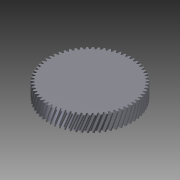
# Autodesk Inventor part: LargeGear
Saved by Autodesk Inventor 2012 (Build 160160000, 160)
## iProperties
Created: 2011-10-22
Part Number: LargeGear
Material: Steel
Document SubType Name: Modeling
Designer: KuttaA
Categories: <?xml version="1.0" encoding="UTF-16"?> <MemberInstance><Categories><FamilyTemplate><FamilyTemplateParameter ValueType="xs:double" Id="1" ObjectReferenceKey="da_z" ObjectType="kUserParameterObject"/><FamilyTemplateParameter ValueType="xs:double" Id="2" ObjectReferenceKey="da_b" ObjectType="kUserParameterObject"/><FamilyTemplateParameter ValueType="xs:double" Id="3" ObjectReferenceKey="da_beta" ObjectType="kUserParameterObject"/><FamilyTemplateParameter ValueType="xs:double" Id="4" ObjectReferenceKey="da_da" ObjectType="kUserParameterObject"/><FamilyTemplateParameter ValueType="xs:double" Id="5" ObjectReferenceKey="da_aw" ObjectType="kUserParameterObject"/><FamilyTemplateParameter ValueType="xs:string" Id="6" ObjectReferenceKey="EAIAABAAAACIAQAAAAAAAIAAAAAAAAAA" ObjectType="83910656" SubObjectId="SurfaceGeometry"/></FamilyTemplate><ParamToTemplateMap><ParamToTemplate CategoryParameter="//CategoryParameter[@InternalName='046C89C9-8512-4d59-83FE-43B91F4F132A']" TemplateParameter="1"/><ParamToTemplate CategoryParameter="//CategoryParameter[@InternalName='2552DF32-E462-4b46-AEBF-C6C7768E72AC']" TemplateParameter="2"/><ParamToTemplate CategoryParameter="//CategoryParameter[@InternalName='C9EE641D-15FC-4fae-A226-E94C4372FDD7']" TemplateParameter="3"/><ParamToTemplate><ParamToTemplate CategoryParameter="//CategoryParameter[@InternalName='00B6519A-459B-49c7-AD84-2E56D39A5744']" ConstantValue="-0.014477"/></ParamToTemplate><ParamToTemplate><ParamToTemplate CategoryParameter="//CategoryParameter[@InternalName='04B31F0E-C7A6-4894-AA32-9629BEFACF47']" ConstantValue="1.000000"/></ParamToTemplate><ParamToTemplate><ParamToTemplate CategoryParameter="//CategoryParameter[@InternalName='43CBEC2E-7847-49e7-A936-2F7889FCB2D9']" ConstantValue="0.250000"/></ParamToTemplate><ParamToTemplate><ParamToTemplate CategoryParameter="//CategoryParameter[@InternalName='B1EFC894-105D-4ebd-86BF-FA20ED196853']" ConstantValue="0.302500"/></ParamToTemplate><ParamToTemplate><ParamToTemplate CategoryParameter="//CategoryParameter[@InternalName='51175063-3D10-4879-93E8-6246FE8B403D']" ConstantValue="2060000000.000000"/></ParamToTemplate><ParamToTemplate><ParamToTemplate CategoryParameter="//CategoryParameter[@InternalName='A3A52E27-4454-46a9-B0BD-C932399B70AF']" ConstantValue="0.300000"/></ParamToTemplate><ParamToTemplate><ParamToTemplate CategoryParameter="//CategoryParameter[@InternalName='91B76062-C214-41d9-B1B9-14D2AB99603D']" ConstantValue="0.031750"/></ParamToTemplate><ParamToTemplate><ParamToTemplate CategoryParameter="//CategoryParameter[@InternalName='374E806E-8B8A-4dda-A9AA-1039D6500AD2']" ConstantValue="31.496063"/></ParamToTemplate><ParamToTemplate><ParamToTemplate CategoryParameter="//CategoryParameter[@InternalName='2D373A89-B862-43d6-8D0B-0CBF12AB9F6C']" ConstantValue="0.349066"/></ParamToTemplate><ParamToTemplate CategoryParameter="//CategoryParameter[@InternalName='37777632-D6A2-4fac-9D53-DB8ACD95C989']" TemplateParameter="4"/><ParamToTemplate CategoryParameter="//CategoryParameter[@InternalName='FD1017F1-B727-4f7e-9707-0F86F1FF9423']" TemplateParameter="5"/><ParamToTemplate><ParamToTemplate CategoryParameter="//CategoryParameter[@InternalName='9E1B4470-B2D3-4ff1-B813-535BB4CDF51A']" ConstantValue="3520000.000000"/></ParamToTemplate><ParamToTemplate><ParamToTemplate CategoryParameter="//CategoryParameter[@InternalName='F8452263-BFF6-458c-9FB1-07C4B99E95CD']" ConstantValue="11400000.000000"/></ParamToTemplate><ParamToTemplate><ParamToTemplate CategoryParameter="//CategoryParameter[@InternalName='3E3BB259-FD49-497f-8171-6EBC954A3479']" ConstantValue="2.000000"/></ParamToTemplate><ParamToTemplate CategoryParameter="//CategoryParameter[@InternalName='27C3BAF2-7550-4e4b-AE2C-0DB134B7D9B7']" TemplateParameter="6"/></ParamToTemplateMap><Category DisplayName="Gear" InternalName="DC85795E-93AB-48d5-8EEE-5A27447B64BD" Mnemonic="Gear"><CategoryParameter DisplayName="z" InternalName="046C89C9-8512-4d59-83FE-43B91F4F132A" Mnemonic="z"/><CategoryParameter DisplayName="b" InternalName="2552DF32-E462-4b46-AEBF-C6C7768E72AC" Mnemonic="b"/><CategoryParameter DisplayName="||b|" InternalName="C9EE641D-15FC-4fae-A226-E94C4372FDD7" Mnemonic="beta"/><CategoryParameter DisplayName="x" InternalName="00B6519A-459B-49c7-AD84-2E56D39A5744" Mnemonic="x"/><CategoryParameter DisplayName="a*" InternalName="04B31F0E-C7A6-4894-AA32-9629BEFACF47" Mnemonic="a"/><CategoryParameter DisplayName="c*" InternalName="43CBEC2E-7847-49e7-A936-2F7889FCB2D9" Mnemonic="c"/><CategoryParameter DisplayName="r|.f|*" InternalName="B1EFC894-105D-4ebd-86BF-FA20ED196853" Mnemonic="rf"/><CategoryParameter DisplayName="E" InternalName="51175063-3D10-4879-93E8-6246FE8B403D" Mnemonic="E"/><CategoryParameter DisplayName="||m|" InternalName="A3A52E27-4454-46a9-B0BD-C932399B70AF" Mnemonic="mi"/><Category DisplayName="SpurGear" InternalName="26C5A22E-A91E-4dfd-A3B3-23CCAFAE1764" Mnemonic="SpurGear"><CategoryParameter DisplayName="m" InternalName="91B76062-C214-41d9-B1B9-14D2AB99603D" Mnemonic="m"/><CategoryParameter DisplayName="P" InternalName="374E806E-8B8A-4dda-A9AA-1039D6500AD2" Mnemonic="PP"/><CategoryParameter DisplayName="||a|" InternalName="2D373A89-B862-43d6-8D0B-0CBF12AB9F6C" Mnemonic="alpha"/><CategoryParameter DisplayName="d|.a|" InternalName="37777632-D6A2-4fac-9D53-DB8ACD95C989" Mnemonic="da"/><CategoryParameter DisplayName="a|.w|" InternalName="FD1017F1-B727-4f7e-9707-0F86F1FF9423" Mnemonic="aw"/><CategoryParameter DisplayName="||s||.Flim|" InternalName="9E1B4470-B2D3-4ff1-B813-535BB4CDF51A" Mnemonic="sFlim"/><CategoryParameter DisplayName="||s||.Hlim|" InternalName="F8452263-BFF6-458c-9FB1-07C4B99E95CD" Mnemonic="sHlim"/><CategoryParameter DisplayName="type" InternalName="3E3BB259-FD49-497f-8171-6EBC954A3479" Mnemonic="type"/><CategoryParameter DisplayName="PitchDiameter" InternalName="27C3BAF2-7550-4e4b-AE2C-0DB134B7D9B7" Mnemonic="IDS_PITCHDIAM"/></Category></Category></Categories></MemberInstance>
Density: 1 g/cm^3
CustomPartVersion: 1
Author: KuttaA
Autodesk Inventor part; units mm, degrees
ref_plane "YZ Plane" through (0, 0, 0) normal (1, 0, 0) x (0, 1, 0)
ref_plane "XZ Plane" through (0, 0, 0) normal (0, 1, 0) x (-1, 0, 0)
ref_plane "XY Plane" through (0, 0, 0) normal (0, 0, 1) x (1, 0, 0)
sketch "Sketch1" plane through (0, 0, 0) normal (0, 0, 1) x (1, 0, 0)
  circle A0 centre (0, 0) radius 10.956
  dimension "d0" = 21.912
  constraints: 1 centre point
  measures "d0" diameter of A0
extrude "Extrusion1" add sketch "Sketch1" along normal blind 4
ref_plane "Work Plane2" through (0, 0, 2) normal (0, 0, 1) x (1, 0, 0)
sketch "Sketch2" plane through (0, 0, 0) normal (0, 0, -1) x (-1, 0, 0)
  circle A0 centre (0, 0) radius 10.956 projected
  circle A1 centre (0, 0) radius 10.6404
  dimension "d3" = 21.2808
  constraints: 1 centre point, 1 coincident
  measures "d3" diameter of A1
surface extrude "Pitch Diameter" sketch "Sketch2" against normal through all shown no curves A1
ref_plane "Work Plane8" through (0, 0, 0) normal (0.9987569, 0.0498459, 0) x (0, 0, 1)
ref_plane "Work Plane9" through (0, 0, 0) normal (1, 0, 0) x (0, 1, 0)
spur gear teeth "Spur Gear" teeth 63 pitch diameter 21.2862 tip diameter 21.912 root diameter 20.4833 face width 4 helix angle 20 hand right start plane through (0, 0, 0) normal (0, 0, -1) x (-1, 0, 0)
sketch "Sketch3" plane through (0, 0, 4) normal (0, 0, 1) x (1, 0, 0)
  spline S0 degree 3 poles (1.3727, 6.9012) (1.3552, 7.1549) (1.3106, 7.4067) (1.2398, 7.651) knots 0 0 0 0 1 1 1 1 construction
  arc A0 (1.2398, 7.651) -> (0.9659, 7.6904) centre (0, 0) ccw construction
  spline S1 degree 3 poles (0.9659, 7.6904) (0.8292, 7.4759) (0.7154, 7.2469) (0.6272, 7.0084) knots 0 0 0 0 1 1 1 1 construction
  spline S2 degree 3 poles (0.6272, 7.0084) (0.5438, 7.0159) (0.4602, 7.0218) (0.3766, 7.0263) knots 0 0 0 0 1 1 1 1 construction
  spline S3 degree 3 poles (0.3766, 7.0263) (0.3232, 7.2749) (0.2432, 7.5179) (0.1383, 7.7495) knots 0 0 0 0 1 1 1 1 construction
  arc A1 (0.1383, 7.7495) -> (-0.1383, 7.7495) centre (0, 0) ccw construction
  spline S4 degree 3 poles (-0.1383, 7.7495) (-0.2432, 7.5179) (-0.3232, 7.2749) (-0.3766, 7.0263) knots 0 0 0 0 1 1 1 1 construction
  spline S5 degree 3 poles (-0.3766, 7.0263) (-0.4602, 7.0218) (-0.5438, 7.0159) (-0.6272, 7.0084) knots 0 0 0 0 1 1 1 1 construction
  spline S6 degree 3 poles (-0.6272, 7.0084) (-0.7154, 7.2469) (-0.8292, 7.4759) (-0.9659, 7.6904) knots 0 0 0 0 1 1 1 1 construction
  arc A2 (-0.9659, 7.6904) -> (-1.2398, 7.651) centre (0, 0) ccw construction
  spline S7 degree 3 poles (-1.2398, 7.651) (-1.3106, 7.4067) (-1.3552, 7.1549) (-1.3727, 6.9012) knots 0 0 0 0 1 1 1 1 construction
  spline S8 degree 3 poles (-1.3727, 6.9012) (-1.4549, 6.8849) (-1.5367, 6.8671) (-1.6182, 6.8478) knots 0 0 0 0 1 1 1 1 construction
  spline S9 degree 3 poles (-1.6182, 6.8478) (-1.7395, 7.0713) (-1.8847, 7.2818) (-2.0506, 7.4746) knots 0 0 0 0 1 1 1 1 construction
  arc A3 (-2.0506, 7.4746) -> (-2.316, 7.3967) centre (0, 0) ccw construction
  spline S10 degree 3 poles (-2.316, 7.3967) (-2.3513, 7.1448) (-2.3597, 6.8892) (-2.3409, 6.6356) knots 0 0 0 0 1 1 1 1 construction
  spline S11 degree 3 poles (-2.3409, 6.6356) (-2.4199, 6.6077) (-2.4983, 6.5785) (-2.5763, 6.5478) knots 0 0 0 0 1 1 1 1 construction
  spline S12 degree 3 poles (-2.5763, 6.5478) (-2.7281, 6.7518) (-2.9018, 6.9395) (-3.0934, 7.1067) knots 0 0 0 0 1 1 1 1 construction
  arc A4 (-3.0934, 7.1067) -> (-3.3451, 6.9918) centre (0, 0) ccw construction
  spline S13 degree 3 poles (-3.3451, 6.9918) (-3.3442, 6.7375) (-3.3161, 6.4833) (-3.2614, 6.2349) knots 0 0 0 0 1 1 1 1 construction
  spline S14 degree 3 poles (-3.2614, 6.2349) (-3.3356, 6.1961) (-3.4091, 6.156) (-3.4819, 6.1145) knots 0 0 0 0 1 1 1 1 construction
  spline S15 degree 3 poles (-3.4819, 6.1145) (-3.6612, 6.2948) (-3.8599, 6.4559) (-4.0733, 6.5941) knots 0 0 0 0 1 1 1 1 construction
  arc A5 (-4.0733, 6.5941) -> (-4.3061, 6.4445) centre (0, 0) ccw construction
  spline S16 degree 3 poles (-4.3061, 6.4445) (-4.269, 6.193) (-4.205, 5.9453) (-4.1155, 5.7073) knots 0 0 0 0 1 1 1 1 construction
  spline S17 degree 3 poles (-4.1155, 5.7073) (-4.1835, 5.6583) (-4.2505, 5.6081) (-4.3166, 5.5568) knots 0 0 0 0 1 1 1 1 construction
  spline S18 degree 3 poles (-4.3166, 5.5568) (-4.5198, 5.7097) (-4.7394, 5.8409) (-4.9703, 5.9473) knots 0 0 0 0 1 1 1 1 construction
  arc A6 (-4.9703, 5.9473) -> (-5.1794, 5.7661) centre (0, 0) ccw construction
  spline S19 degree 3 poles (-5.1794, 5.7661) (-5.1069, 5.5224) (-5.0083, 5.2864) (-4.8859, 5.0635) knots 0 0 0 0 1 1 1 1 construction
  spline S20 degree 3 poles (-4.8859, 5.0635) (-4.9461, 5.0054) (-5.0054, 4.9461) (-5.0635, 4.8859) knots 0 0 0 0 1 1 1 1 construction
  spline S21 degree 3 poles (-5.0635, 4.8859) (-5.2864, 5.0083) (-5.5224, 5.1069) (-5.7661, 5.1794) knots 0 0 0 0 1 1 1 1 construction
  arc A7 (-5.7661, 5.1794) -> (-5.9473, 4.9703) centre (0, 0) ccw construction
  spline S22 degree 3 poles (-5.9473, 4.9703) (-5.8409, 4.7394) (-5.7097, 4.5198) (-5.5568, 4.3166) knots 0 0 0 0 1 1 1 1 construction
  spline S23 degree 3 poles (-5.5568, 4.3166) (-5.6081, 4.2505) (-5.6583, 4.1835) (-5.7073, 4.1155) knots 0 0 0 0 1 1 1 1 construction
  spline S24 degree 3 poles (-5.7073, 4.1155) (-5.9453, 4.205) (-6.193, 4.269) (-6.4445, 4.3061) knots 0 0 0 0 1 1 1 1 construction
  arc A8 (-6.4445, 4.3061) -> (-6.5941, 4.0733) centre (0, 0) ccw construction
  spline S25 degree 3 poles (-6.5941, 4.0733) (-6.4559, 3.8599) (-6.2948, 3.6612) (-6.1145, 3.4819) knots 0 0 0 0 1 1 1 1 construction
  spline S26 degree 3 poles (-6.1145, 3.4819) (-6.156, 3.4091) (-6.1961, 3.3356) (-6.2349, 3.2614) knots 0 0 0 0 1 1 1 1 construction
  spline S27 degree 3 poles (-6.2349, 3.2614) (-6.4833, 3.3161) (-6.7375, 3.3442) (-6.9918, 3.3451) knots 0 0 0 0 1 1 1 1 construction
  arc A9 (-6.9918, 3.3451) -> (-7.1067, 3.0934) centre (0, 0) ccw construction
  spline S28 degree 3 poles (-7.1067, 3.0934) (-6.9395, 2.9018) (-6.7518, 2.7281) (-6.5478, 2.5763) knots 0 0 0 0 1 1 1 1 construction
  spline S29 degree 3 poles (-6.5478, 2.5763) (-6.5785, 2.4983) (-6.6077, 2.4199) (-6.6356, 2.3409) knots 0 0 0 0 1 1 1 1 construction
  spline S30 degree 3 poles (-6.6356, 2.3409) (-6.8892, 2.3597) (-7.1448, 2.3513) (-7.3967, 2.316) knots 0 0 0 0 1 1 1 1 construction
  arc A10 (-7.3967, 2.316) -> (-7.4746, 2.0506) centre (0, 0) ccw construction
  spline S31 degree 3 poles (-7.4746, 2.0506) (-7.2818, 1.8847) (-7.0713, 1.7395) (-6.8478, 1.6182) knots 0 0 0 0 1 1 1 1 construction
  spline S32 degree 3 poles (-6.8478, 1.6182) (-6.8671, 1.5367) (-6.8849, 1.4549) (-6.9012, 1.3727) knots 0 0 0 0 1 1 1 1 construction
  spline S33 degree 3 poles (-6.9012, 1.3727) (-7.1549, 1.3552) (-7.4067, 1.3106) (-7.651, 1.2398) knots 0 0 0 0 1 1 1 1 construction
  arc A11 (-7.651, 1.2398) -> (-7.6904, 0.9659) centre (0, 0) ccw construction
  spline S34 degree 3 poles (-7.6904, 0.9659) (-7.4759, 0.8292) (-7.2469, 0.7154) (-7.0084, 0.6272) knots 0 0 0 0 1 1 1 1 construction
  spline S35 degree 3 poles (-7.0084, 0.6272) (-7.0159, 0.5438) (-7.0218, 0.4602) (-7.0263, 0.3766) knots 0 0 0 0 1 1 1 1 construction
  spline S36 degree 3 poles (-7.0263, 0.3766) (-7.2749, 0.3232) (-7.5179, 0.2432) (-7.7495, 0.1383) knots 0 0 0 0 1 1 1 1 construction
  arc A12 (-7.7495, 0.1383) -> (-7.7495, -0.1383) centre (0, 0) ccw construction
  spline S37 degree 3 poles (-7.7495, -0.1383) (-7.5179, -0.2432) (-7.2749, -0.3232) (-7.0263, -0.3766) knots 0 0 0 0 1 1 1 1 construction
  spline S38 degree 3 poles (-7.0263, -0.3766) (-7.0218, -0.4602) (-7.0159, -0.5438) (-7.0084, -0.6272) knots 0 0 0 0 1 1 1 1 construction
  spline S39 degree 3 poles (-7.0084, -0.6272) (-7.2469, -0.7154) (-7.4759, -0.8292) (-7.6904, -0.9659) knots 0 0 0 0 1 1 1 1 construction
  arc A13 (-7.6904, -0.9659) -> (-7.651, -1.2398) centre (0, 0) ccw construction
  spline S40 degree 3 poles (-7.651, -1.2398) (-7.4067, -1.3106) (-7.1549, -1.3552) (-6.9012, -1.3727) knots 0 0 0 0 1 1 1 1 construction
  spline S41 degree 3 poles (-6.9012, -1.3727) (-6.8849, -1.4549) (-6.8671, -1.5367) (-6.8478, -1.6182) knots 0 0 0 0 1 1 1 1 construction
  spline S42 degree 3 poles (-6.8478, -1.6182) (-7.0713, -1.7395) (-7.2818, -1.8847) (-7.4746, -2.0506) knots 0 0 0 0 1 1 1 1 construction
  arc A14 (-7.4746, -2.0506) -> (-7.3967, -2.316) centre (0, 0) ccw construction
  spline S43 degree 3 poles (-7.3967, -2.316) (-7.1448, -2.3513) (-6.8892, -2.3597) (-6.6356, -2.3409) knots 0 0 0 0 1 1 1 1 construction
  spline S44 degree 3 poles (-6.6356, -2.3409) (-6.6077, -2.4199) (-6.5785, -2.4983) (-6.5478, -2.5763) knots 0 0 0 0 1 1 1 1 construction
  spline S45 degree 3 poles (-6.5478, -2.5763) (-6.7518, -2.7281) (-6.9395, -2.9018) (-7.1067, -3.0934) knots 0 0 0 0 1 1 1 1 construction
  arc A15 (-7.1067, -3.0934) -> (-6.9918, -3.3451) centre (0, 0) ccw construction
  spline S46 degree 3 poles (-6.9918, -3.3451) (-6.7375, -3.3442) (-6.4833, -3.3161) (-6.2349, -3.2614) knots 0 0 0 0 1 1 1 1 construction
  spline S47 degree 3 poles (-6.2349, -3.2614) (-6.1961, -3.3356) (-6.156, -3.4091) (-6.1145, -3.4819) knots 0 0 0 0 1 1 1 1 construction
  spline S48 degree 3 poles (-6.1145, -3.4819) (-6.2948, -3.6612) (-6.4559, -3.8599) (-6.5941, -4.0733) knots 0 0 0 0 1 1 1 1 construction
  arc A16 (-6.5941, -4.0733) -> (-6.4445, -4.3061) centre (0, 0) ccw construction
  spline S49 degree 3 poles (-6.4445, -4.3061) (-6.193, -4.269) (-5.9453, -4.205) (-5.7073, -4.1155) knots 0 0 0 0 1 1 1 1 construction
  spline S50 degree 3 poles (-5.7073, -4.1155) (-5.6583, -4.1835) (-5.6081, -4.2505) (-5.5568, -4.3166) knots 0 0 0 0 1 1 1 1 construction
  spline S51 degree 3 poles (-5.5568, -4.3166) (-5.7097, -4.5198) (-5.8409, -4.7394) (-5.9473, -4.9703) knots 0 0 0 0 1 1 1 1 construction
  arc A17 (-5.9473, -4.9703) -> (-5.7661, -5.1794) centre (0, 0) ccw construction
  spline S52 degree 3 poles (-5.7661, -5.1794) (-5.5224, -5.1069) (-5.2864, -5.0083) (-5.0635, -4.8859) knots 0 0 0 0 1 1 1 1 construction
  spline S53 degree 3 poles (-5.0635, -4.8859) (-5.0054, -4.9461) (-4.9461, -5.0054) (-4.8859, -5.0635) knots 0 0 0 0 1 1 1 1 construction
  spline S54 degree 3 poles (-4.8859, -5.0635) (-5.0083, -5.2864) (-5.1069, -5.5224) (-5.1794, -5.7661) knots 0 0 0 0 1 1 1 1 construction
  arc A18 (-5.1794, -5.7661) -> (-4.9703, -5.9473) centre (0, 0) ccw construction
  spline S55 degree 3 poles (-4.9703, -5.9473) (-4.7394, -5.8409) (-4.5198, -5.7097) (-4.3166, -5.5568) knots 0 0 0 0 1 1 1 1 construction
  spline S56 degree 3 poles (-4.3166, -5.5568) (-4.2505, -5.6081) (-4.1835, -5.6583) (-4.1155, -5.7073) knots 0 0 0 0 1 1 1 1 construction
  spline S57 degree 3 poles (-4.1155, -5.7073) (-4.205, -5.9453) (-4.269, -6.193) (-4.3061, -6.4445) knots 0 0 0 0 1 1 1 1 construction
  arc A19 (-4.3061, -6.4445) -> (-4.0733, -6.5941) centre (0, 0) ccw construction
  spline S58 degree 3 poles (-4.0733, -6.5941) (-3.8599, -6.4559) (-3.6612, -6.2948) (-3.4819, -6.1145) knots 0 0 0 0 1 1 1 1 construction
  spline S59 degree 3 poles (-3.4819, -6.1145) (-3.4091, -6.156) (-3.3356, -6.1961) (-3.2614, -6.2349) knots 0 0 0 0 1 1 1 1 construction
  spline S60 degree 3 poles (-3.2614, -6.2349) (-3.3161, -6.4833) (-3.3442, -6.7375) (-3.3451, -6.9918) knots 0 0 0 0 1 1 1 1 construction
  arc A20 (-3.3451, -6.9918) -> (-3.0934, -7.1067) centre (0, 0) ccw construction
  spline S61 degree 3 poles (-3.0934, -7.1067) (-2.9018, -6.9395) (-2.7281, -6.7518) (-2.5763, -6.5478) knots 0 0 0 0 1 1 1 1 construction
  spline S62 degree 3 poles (-2.5763, -6.5478) (-2.4983, -6.5785) (-2.4199, -6.6077) (-2.3409, -6.6356) knots 0 0 0 0 1 1 1 1 construction
  spline S63 degree 3 poles (-2.3409, -6.6356) (-2.3597, -6.8892) (-2.3513, -7.1448) (-2.316, -7.3967) knots 0 0 0 0 1 1 1 1 construction
  arc A21 (-2.316, -7.3967) -> (-2.0506, -7.4746) centre (0, 0) ccw construction
  spline S64 degree 3 poles (-2.0506, -7.4746) (-1.8847, -7.2818) (-1.7395, -7.0713) (-1.6182, -6.8478) knots 0 0 0 0 1 1 1 1 construction
  spline S65 degree 3 poles (-1.6182, -6.8478) (-1.5367, -6.8671) (-1.4549, -6.8849) (-1.3727, -6.9012) knots 0 0 0 0 1 1 1 1 construction
  spline S66 degree 3 poles (-1.3727, -6.9012) (-1.3552, -7.1549) (-1.3106, -7.4067) (-1.2398, -7.651) knots 0 0 0 0 1 1 1 1 construction
  arc A22 (-1.2398, -7.651) -> (-0.9659, -7.6904) centre (0, 0) ccw construction
  spline S67 degree 3 poles (-0.9659, -7.6904) (-0.8292, -7.4759) (-0.7154, -7.2469) (-0.6272, -7.0084) knots 0 0 0 0 1 1 1 1 construction
  spline S68 degree 3 poles (-0.6272, -7.0084) (-0.5438, -7.0159) (-0.4602, -7.0218) (-0.3766, -7.0263) knots 0 0 0 0 1 1 1 1 construction
  spline S69 degree 3 poles (-0.3766, -7.0263) (-0.3232, -7.2749) (-0.2432, -7.5179) (-0.1383, -7.7495) knots 0 0 0 0 1 1 1 1 construction
  arc A23 (-0.1383, -7.7495) -> (0.1383, -7.7495) centre (0, 0) ccw construction
  spline S70 degree 3 poles (0.1383, -7.7495) (0.2432, -7.5179) (0.3232, -7.2749) (0.3766, -7.0263) knots 0 0 0 0 1 1 1 1 construction
  spline S71 degree 3 poles (0.3766, -7.0263) (0.4602, -7.0218) (0.5438, -7.0159) (0.6272, -7.0084) knots 0 0 0 0 1 1 1 1 construction
  spline S72 degree 3 poles (0.6272, -7.0084) (0.7154, -7.2469) (0.8292, -7.4759) (0.9659, -7.6904) knots 0 0 0 0 1 1 1 1 construction
  arc A24 (0.9659, -7.6904) -> (1.2398, -7.651) centre (0, 0) ccw construction
  spline S73 degree 3 poles (1.2398, -7.651) (1.3106, -7.4067) (1.3552, -7.1549) (1.3727, -6.9012) knots 0 0 0 0 1 1 1 1 construction
  spline S74 degree 3 poles (1.3727, -6.9012) (1.4549, -6.8849) (1.5367, -6.8671) (1.6182, -6.8478) knots 0 0 0 0 1 1 1 1 construction
  spline S75 degree 3 poles (1.6182, -6.8478) (1.7395, -7.0713) (1.8847, -7.2818) (2.0506, -7.4746) knots 0 0 0 0 1 1 1 1 construction
  arc A25 (2.0506, -7.4746) -> (2.316, -7.3967) centre (0, 0) ccw construction
  spline S76 degree 3 poles (2.316, -7.3967) (2.3513, -7.1448) (2.3597, -6.8892) (2.3409, -6.6356) knots 0 0 0 0 1 1 1 1 construction
  spline S77 degree 3 poles (2.3409, -6.6356) (2.4199, -6.6077) (2.4983, -6.5785) (2.5763, -6.5478) knots 0 0 0 0 1 1 1 1 construction
  spline S78 degree 3 poles (2.5763, -6.5478) (2.7281, -6.7518) (2.9018, -6.9395) (3.0934, -7.1067) knots 0 0 0 0 1 1 1 1 construction
  arc A26 (3.0934, -7.1067) -> (3.3451, -6.9918) centre (0, 0) ccw construction
  spline S79 degree 3 poles (3.3451, -6.9918) (3.3442, -6.7375) (3.3161, -6.4833) (3.2614, -6.2349) knots 0 0 0 0 1 1 1 1 construction
  spline S80 degree 3 poles (3.2614, -6.2349) (3.3356, -6.1961) (3.4091, -6.156) (3.4819, -6.1145) knots 0 0 0 0 1 1 1 1 construction
  spline S81 degree 3 poles (3.4819, -6.1145) (3.6612, -6.2948) (3.8599, -6.4559) (4.0733, -6.5941) knots 0 0 0 0 1 1 1 1 construction
  arc A27 (4.0733, -6.5941) -> (4.3061, -6.4445) centre (0, 0) ccw construction
  spline S82 degree 3 poles (4.3061, -6.4445) (4.269, -6.193) (4.205, -5.9453) (4.1155, -5.7073) knots 0 0 0 0 1 1 1 1 construction
  spline S83 degree 3 poles (4.1155, -5.7073) (4.1835, -5.6583) (4.2505, -5.6081) (4.3166, -5.5568) knots 0 0 0 0 1 1 1 1 construction
  spline S84 degree 3 poles (4.3166, -5.5568) (4.5198, -5.7097) (4.7394, -5.8409) (4.9703, -5.9473) knots 0 0 0 0 1 1 1 1 construction
  arc A28 (4.9703, -5.9473) -> (5.1794, -5.7661) centre (0, 0) ccw construction
  spline S85 degree 3 poles (5.1794, -5.7661) (5.1069, -5.5224) (5.0083, -5.2864) (4.8859, -5.0635) knots 0 0 0 0 1 1 1 1 construction
  spline S86 degree 3 poles (4.8859, -5.0635) (4.9461, -5.0054) (5.0054, -4.9461) (5.0635, -4.8859) knots 0 0 0 0 1 1 1 1 construction
  spline S87 degree 3 poles (5.0635, -4.8859) (5.2864, -5.0083) (5.5224, -5.1069) (5.7661, -5.1794) knots 0 0 0 0 1 1 1 1 construction
  arc A29 (5.7661, -5.1794) -> (5.9473, -4.9703) centre (0, 0) ccw construction
  spline S88 degree 3 poles (5.9473, -4.9703) (5.8409, -4.7394) (5.7097, -4.5198) (5.5568, -4.3166) knots 0 0 0 0 1 1 1 1 construction
  spline S89 degree 3 poles (5.5568, -4.3166) (5.6081, -4.2505) (5.6583, -4.1835) (5.7073, -4.1155) knots 0 0 0 0 1 1 1 1 construction
  spline S90 degree 3 poles (5.7073, -4.1155) (5.9453, -4.205) (6.193, -4.269) (6.4445, -4.3061) knots 0 0 0 0 1 1 1 1 construction
  arc A30 (6.4445, -4.3061) -> (6.5941, -4.0733) centre (0, 0) ccw construction
  spline S91 degree 3 poles (6.5941, -4.0733) (6.4559, -3.8599) (6.2948, -3.6612) (6.1145, -3.4819) knots 0 0 0 0 1 1 1 1 construction
  spline S92 degree 3 poles (6.1145, -3.4819) (6.156, -3.4091) (6.1961, -3.3356) (6.2349, -3.2614) knots 0 0 0 0 1 1 1 1 construction
  spline S93 degree 3 poles (6.2349, -3.2614) (6.4833, -3.3161) (6.7375, -3.3442) (6.9918, -3.3451) knots 0 0 0 0 1 1 1 1 construction
  arc A31 (6.9918, -3.3451) -> (7.1067, -3.0934) centre (0, 0) ccw construction
  spline S94 degree 3 poles (7.1067, -3.0934) (6.9395, -2.9018) (6.7518, -2.7281) (6.5478, -2.5763) knots 0 0 0 0 1 1 1 1 construction
  spline S95 degree 3 poles (6.5478, -2.5763) (6.5785, -2.4983) (6.6077, -2.4199) (6.6356, -2.3409) knots 0 0 0 0 1 1 1 1 construction
  spline S96 degree 3 poles (6.6356, -2.3409) (6.8892, -2.3597) (7.1448, -2.3513) (7.3967, -2.316) knots 0 0 0 0 1 1 1 1 construction
  arc A32 (7.3967, -2.316) -> (7.4746, -2.0506) centre (0, 0) ccw construction
  spline S97 degree 3 poles (7.4746, -2.0506) (7.2818, -1.8847) (7.0713, -1.7395) (6.8478, -1.6182) knots 0 0 0 0 1 1 1 1 construction
  spline S98 degree 3 poles (6.8478, -1.6182) (6.8671, -1.5367) (6.8849, -1.4549) (6.9012, -1.3727) knots 0 0 0 0 1 1 1 1 construction
  spline S99 degree 3 poles (6.9012, -1.3727) (7.1549, -1.3552) (7.4067, -1.3106) (7.651, -1.2398) knots 0 0 0 0 1 1 1 1 construction
  arc A33 (7.651, -1.2398) -> (7.6904, -0.9659) centre (0, 0) ccw construction
  spline S100 degree 3 poles (7.6904, -0.9659) (7.4759, -0.8292) (7.2469, -0.7154) (7.0084, -0.6272) knots 0 0 0 0 1 1 1 1 construction
  spline S101 degree 3 poles (7.0084, -0.6272) (7.0159, -0.5438) (7.0218, -0.4602) (7.0263, -0.3766) knots 0 0 0 0 1 1 1 1 construction
  spline S102 degree 3 poles (7.0263, -0.3766) (7.2749, -0.3232) (7.5179, -0.2432) (7.7495, -0.1383) knots 0 0 0 0 1 1 1 1 construction
  arc A34 (7.7495, -0.1383) -> (7.7495, 0.1383) centre (0, 0) ccw construction
  spline S103 degree 3 poles (7.7495, 0.1383) (7.5179, 0.2432) (7.2749, 0.3232) (7.0263, 0.3766) knots 0 0 0 0 1 1 1 1 construction
  spline S104 degree 3 poles (7.0263, 0.3766) (7.0218, 0.4602) (7.0159, 0.5438) (7.0084, 0.6272) knots 0 0 0 0 1 1 1 1 construction
  spline S105 degree 3 poles (7.0084, 0.6272) (7.2469, 0.7154) (7.4759, 0.8292) (7.6904, 0.9659) knots 0 0 0 0 1 1 1 1 construction
  arc A35 (7.6904, 0.9659) -> (7.651, 1.2398) centre (0, 0) ccw construction
  spline S106 degree 3 poles (7.651, 1.2398) (7.4067, 1.3106) (7.1549, 1.3552) (6.9012, 1.3727) knots 0 0 0 0 1 1 1 1 construction
  spline S107 degree 3 poles (6.9012, 1.3727) (6.8849, 1.4549) (6.8671, 1.5367) (6.8478, 1.6182) knots 0 0 0 0 1 1 1 1 construction
  spline S108 degree 3 poles (6.8478, 1.6182) (7.0713, 1.7395) (7.2818, 1.8847) (7.4746, 2.0506) knots 0 0 0 0 1 1 1 1 construction
  arc A36 (7.4746, 2.0506) -> (7.3967, 2.316) centre (0, 0) ccw construction
  spline S109 degree 3 poles (7.3967, 2.316) (7.1448, 2.3513) (6.8892, 2.3597) (6.6356, 2.3409) knots 0 0 0 0 1 1 1 1 construction
  spline S110 degree 3 poles (6.6356, 2.3409) (6.6077, 2.4199) (6.5785, 2.4983) (6.5478, 2.5763) knots 0 0 0 0 1 1 1 1 construction
  spline S111 degree 3 poles (6.5478, 2.5763) (6.7518, 2.7281) (6.9395, 2.9018) (7.1067, 3.0934) knots 0 0 0 0 1 1 1 1 construction
  arc A37 (7.1067, 3.0934) -> (6.9918, 3.3451) centre (0, 0) ccw construction
  spline S112 degree 3 poles (6.9918, 3.3451) (6.7375, 3.3442) (6.4833, 3.3161) (6.2349, 3.2614) knots 0 0 0 0 1 1 1 1 construction
  spline S113 degree 3 poles (6.2349, 3.2614) (6.1961, 3.3356) (6.156, 3.4091) (6.1145, 3.4819) knots 0 0 0 0 1 1 1 1 construction
  spline S114 degree 3 poles (6.1145, 3.4819) (6.2948, 3.6612) (6.4559, 3.8599) (6.5941, 4.0733) knots 0 0 0 0 1 1 1 1 construction
  arc A38 (6.5941, 4.0733) -> (6.4445, 4.3061) centre (0, 0) ccw construction
  spline S115 degree 3 poles (6.4445, 4.3061) (6.193, 4.269) (5.9453, 4.205) (5.7073, 4.1155) knots 0 0 0 0 1 1 1 1 construction
  spline S116 degree 3 poles (5.7073, 4.1155) (5.6583, 4.1835) (5.6081, 4.2505) (5.5568, 4.3166) knots 0 0 0 0 1 1 1 1 construction
  spline S117 degree 3 poles (5.5568, 4.3166) (5.7097, 4.5198) (5.8409, 4.7394) (5.9473, 4.9703) knots 0 0 0 0 1 1 1 1 construction
  arc A39 (5.9473, 4.9703) -> (5.7661, 5.1794) centre (0, 0) ccw construction
  spline S118 degree 3 poles (5.7661, 5.1794) (5.5224, 5.1069) (5.2864, 5.0083) (5.0635, 4.8859) knots 0 0 0 0 1 1 1 1 construction
  spline S119 degree 3 poles (5.0635, 4.8859) (5.0054, 4.9461) (4.9461, 5.0054) (4.8859, 5.0635) knots 0 0 0 0 1 1 1 1 construction
  spline S120 degree 3 poles (4.8859, 5.0635) (5.0083, 5.2864) (5.1069, 5.5224) (5.1794, 5.7661) knots 0 0 0 0 1 1 1 1 construction
  arc A40 (5.1794, 5.7661) -> (4.9703, 5.9473) centre (0, 0) ccw construction
  spline S121 degree 3 poles (4.9703, 5.9473) (4.7394, 5.8409) (4.5198, 5.7097) (4.3166, 5.5568) knots 0 0 0 0 1 1 1 1 construction
  spline S122 degree 3 poles (4.3166, 5.5568) (4.2505, 5.6081) (4.1835, 5.6583) (4.1155, 5.7073) knots 0 0 0 0 1 1 1 1 construction
  spline S123 degree 3 poles (4.1155, 5.7073) (4.205, 5.9453) (4.269, 6.193) (4.3061, 6.4445) knots 0 0 0 0 1 1 1 1 construction
  arc A41 (4.3061, 6.4445) -> (4.0733, 6.5941) centre (0, 0) ccw construction
  spline S124 degree 3 poles (4.0733, 6.5941) (3.8599, 6.4559) (3.6612, 6.2948) (3.4819, 6.1145) knots 0 0 0 0 1 1 1 1 construction
  spline S125 degree 3 poles (3.4819, 6.1145) (3.4091, 6.156) (3.3356, 6.1961) (3.2614, 6.2349) knots 0 0 0 0 1 1 1 1 construction
  spline S126 degree 3 poles (3.2614, 6.2349) (3.3161, 6.4833) (3.3442, 6.7375) (3.3451, 6.9918) knots 0 0 0 0 1 1 1 1 construction
  arc A42 (3.3451, 6.9918) -> (3.0934, 7.1067) centre (0, 0) ccw construction
  spline S127 degree 3 poles (3.0934, 7.1067) (2.9018, 6.9395) (2.7281, 6.7518) (2.5763, 6.5478) knots 0 0 0 0 1 1 1 1 construction
  spline S128 degree 3 poles (2.5763, 6.5478) (2.4983, 6.5785) (2.4199, 6.6077) (2.3409, 6.6356) knots 0 0 0 0 1 1 1 1 construction
  spline S129 degree 3 poles (2.3409, 6.6356) (2.3597, 6.8892) (2.3513, 7.1448) (2.316, 7.3967) knots 0 0 0 0 1 1 1 1 construction
  arc A43 (2.316, 7.3967) -> (2.0506, 7.4746) centre (0, 0) ccw construction
  spline S130 degree 3 poles (2.0506, 7.4746) (1.8847, 7.2818) (1.7395, 7.0713) (1.6182, 6.8478) knots 0 0 0 0 1 1 1 1 construction
  spline S131 degree 3 poles (1.6182, 6.8478) (1.5367, 6.8671) (1.4549, 6.8849) (1.3727, 6.9012) knots 0 0 0 0 1 1 1 1 construction
  circle A44 centre (0, 0) radius 7.0364
  circle A45 centre (0, 0) radius 3
  point P0 (0, 0)
  constraints: 1 coincident, 3 other
extrude "Extrusion2" add sketch "Sketch3" along normal blind 2 contours A44 | A45
equation "\"d0\" = da_da"
equation "\"d1\" = da_b"
equation "\"d3\" = da_dw"
equation "\"d16\" = da_aw"
equation "\"d43\" = da_aw"
equation "\"d46\" = da_aw"
equation "\"da_da\" = 21.912015"
equation "\"da_b\" = 4"
equation "\"da_dw\" = 21.280799"
equation "\"da_aw\" = 18.071789"
body "Solid1"
body "Srf1"
